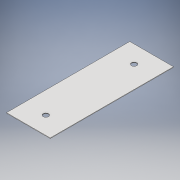
# Autodesk Inventor part: Molex Flexible GNSS Antenna
Saved by Autodesk Inventor 2019 (Build 230136000, 136)
## iProperties
Created: 2020-08-03
Part Number: Molex Flexible GNSS Antenna
Material: Generic
Document SubType Name: Modeling
Designer: james
Density: 1 g/cm^3
Appearance: Default(1)
Author: james
Autodesk Inventor part; units mm, degrees
ref_plane "YZ Plane" through (0, 0, 0) normal (1, 0, 0) x (0, 1, 0)
ref_plane "XZ Plane" through (0, 0, 0) normal (0, 1, 0) x (-1, 0, 0)
ref_plane "XY Plane" through (0, 0, 0) normal (0, 0, 1) x (1, 0, 0)
sketch "Sketch1" plane through (0, 0, 0) normal (0, 1, 0) x (-1, 0, 0)
  line L0 (19.7747, 24.136) -> (-0.2253, 24.136)
  line L1 (-0.2253, 24.136) -> (-0.2253, -32.264)
  line L2 (-0.2253, -32.264) -> (19.7747, -32.264)
  line L3 (19.7747, -32.264) -> (19.7747, 24.136)
  point P0 (0, 0)
  dimension "d0" = 56.4
  dimension "d1" = 20
  constraints: 8 end point, 2 parallel, 1 horizontal, 1 perpendicular
  measures "d0" distance of L2.end L0.start
  measures "d1" distance of L0.start L0.end
extrude "Extrusion1" add sketch "Sketch1" along normal blind 0.254
sketch "Sketch2" plane through (0, 0.254, 0) normal (0, 1, 0) x (1, 0, 0)
  line L0 (-19.7747, 32.264) -> (-19.7747, -24.136) projected
  line L1 (-19.7747, -24.136) -> (0.2253, -24.136) projected
  line L2 (0.2253, 32.264) -> (-19.7747, 32.264) projected
  point P0 (0, 0)
  point P1 (-9.7747, -16.136)
  point P2 (-9.7747, 24.264)
  dimension "d4" = 10
  dimension "d5" = 0
  dimension "d6" = 8
  dimension "d7" = 8
  measures "d4" distance from line of L0 point (-9.775, -16.136)
  measures "d5" horizontal distance of point (-9.775, 24.264) point (-9.775, -16.136)
  measures "d6" distance from line of L1 point (-9.775, -16.136)
  measures "d7" distance from line of L2 point (-9.775, 24.264)
hole "Hole1" at (-9.7747, 0.254, 16.136) at (-9.7747, 0.254, -24.264) direction (0, -1, 0) diameter 2.4638 end through all
body "Solid1"
